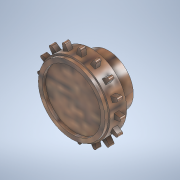
# Autodesk Inventor part: velke_koleso
Saved by Autodesk Inventor 2022 (Build 260153000, 153)
## iProperties
Created: 2021-12-16
Part Number: velke_koleso
Material: Generic
Document SubType Name: Modeling
Designer: MatusBarany
Density: 1 g/cm^3
Appearance: Default
Author: MatusBarany
Autodesk Inventor part; units mm, degrees
ref_plane "YZ Plane" through (0, 0, 0) normal (1, 0, 0) x (0, 1, 0)
ref_plane "XZ Plane" through (0, 0, 0) normal (0, 1, 0) x (-1, 0, 0)
ref_plane "XY Plane" through (0, 0, 0) normal (0, 0, 1) x (1, 0, 0)
sketch "Sketch1" plane through (0, 0, 0) normal (0, 0, 1) x (1, 0, 0)
  circle A0 centre (0, 0) radius 21
  dimension "d0" = 42
  constraints: 1 centre point, 1 coincident
  measures "d0" diameter of A0
extrude "Extrusion1" add sketch "Sketch1" along normal blind 10
sketch "Sketch2" plane through (0, 0, 10) normal (0, 0, 1) x (1, 0, 0)
  circle A0 centre (0, 0) radius 20
  circle A1 centre (0, 0) radius 21 projected
  circle A2 centre (0, 0) radius 17.5
  dimension "d3" = 40
  dimension "d4" = 42
  dimension "d5" = 35
  constraints: 2 centre point, 2 coincident
  measures "d3" diameter of A0
  measures "d4" diameter of A1
  measures "d5" diameter of A2
extrude "Extrusion2" add sketch "Sketch2" along normal blind 2 contours A0
ref_plane "Work Plane1" through (0, 0, 6) normal (0, 0, 1) x (1, 0, 0)
sketch "Sketch3" plane through (0, 0, 6) normal (0, 0, 1) x (1, 0, 0)
  circle A0 centre (0, 0) radius 21 projected
  line L0 (0, 25) -> (0, 21)
  line L1 (0, -30.2358) -> (0, 34.4151) projected
  line L2 (-0.9848, 24.1736) -> (-1.5546, 20.9424)
  arc A1 (0, 25) -> (-0.9848, 24.1736) centre (0, 24) ccw
  line L3 (0.9848, 24.1736) -> (1.5546, 20.9424)
  arc A2 (0.9848, 24.1736) -> (0, 25) centre (0, 24) ccw
  point P0 (1.5546, 20.9424)
  dimension "d12" = 1
  dimension "d14" = 10
  dimension "d15" = 4
  constraints: 6 end point, 6 point on circle, 2 centre point, 2 collinear, 2 symmetric about line, 1 point on line, 1 tangent, 1 vertical, 1 other
  measures "d12" radius of A1
  measures "d14" angle of L2 L0
  measures "d15" distance of L0.start L0.end
extrude "Extrusion3" add sketch "Sketch3" along normal mid plane 3 contours A0 L0 A2 L3 | A0 L2 A1 L0
pattern_circular "Circular Pattern1" count 16 over 360 about axis through (0, 0, -10) along (0, 0, 1) of "Extrusion3"
sketch "Sketch4" plane through (0, 0, 0) normal (0, 0, -1) x (-1, 0, 0)
  circle A0 centre (0, 0) radius 17.5 projected
  circle A1 centre (0, 0) radius 15
  arc A2 (-7.5, 8.0467) -> (7.5, 8.0467) centre (0, 0) ccw
  line L0 (7.5, 8.0467) -> (-7.5, 8.0467)
  dimension "d23" = 22
  dimension "d24" = 30
  dimension "d25" = 15
  constraints: 2 centre point, 2 coincident, 2 end point, 2 point on circle, 1 horizontal
  measures "d23" diameter of A2
  measures "d24" diameter of A1
  measures "d25" distance of L0.start L0.end
extrude "Extrusion4" add sketch "Sketch4" along normal blind 10 contours A1
body "Solid1"
